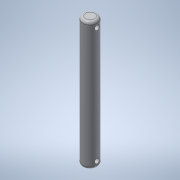
# Autodesk Inventor part: Eixo_16mm
Saved by Autodesk Inventor 2022 (Build 260153000, 153)
## iProperties
Manager: Standard
Created: 2016-02-21
Part Number: Eixo_16mm
Material: SAE 1010/1020
Document SubType Name: Modeling
Designer: Everton
Authority: Rafael Salvador
Manufacturer: Standard
Standards Organization: Custom
Density: 7.86 g/cm^3
Appearance: Steel
Author: Everton
Comments: -
Revision Number: 00
Autodesk Inventor part; units mm, degrees
ref_plane "YZ Plane" through (0, 0, 0) normal (1, 0, 0) x (0, 1, 0)
ref_plane "XZ Plane" through (0, 0, 0) normal (0, 1, 0) x (-1, 0, 0)
ref_plane "XY Plane" through (0, 0, 0) normal (0, 0, 1) x (1, 0, 0)
sketch "Sketch1" plane through (0, 0, 0) normal (0, 0, 1) x (1, 0, 0)
  circle A0 centre (-11.2222, 3.5185) radius 8
  point P0 (0, 0)
  dimension "d0" = 16
  constraints: 1 centre point
  measures "d0" diameter of A0
extrude "Extrusion1" add sketch "Sketch1" along normal blind 140
fillet "Fillet1" radius 3 2 edges at (-19.2222, 3.5185, 140) (-19.2222, 3.5185, 0)
sketch "Sketch2" plane through (0, 0, 0) normal (1, 0, 0) x (0, 1, 0)
  line L0 (-1.4815, 140) -> (8.5185, 140) projected
  line L1 (3.5185, 140) -> (3.5185, 40)
  circle A0 centre (3.5185, 133) radius 2.5
  circle A1 centre (3.5185, 7) radius 2.5
  line L2 (8.5185, 0) -> (-1.4815, 0) projected
  point P0 (0, 0)
  dimension "d4" = 5
  dimension "d5" = 5
  dimension "d6" = 7
  dimension "d10" = 7
  constraints: 2 centre point, 2 end point, 2 point on line, 1 midpoint, 1 vertical
  measures "d4" diameter of A0
  measures "d5" diameter of A1
  measures "d6" distance of L1.start A0.centre
  measures "d10" distance from line of L2 A1.centre
extrude "Extrusion2" cut sketch "Sketch2" against normal blind 100
body "Solid1"
